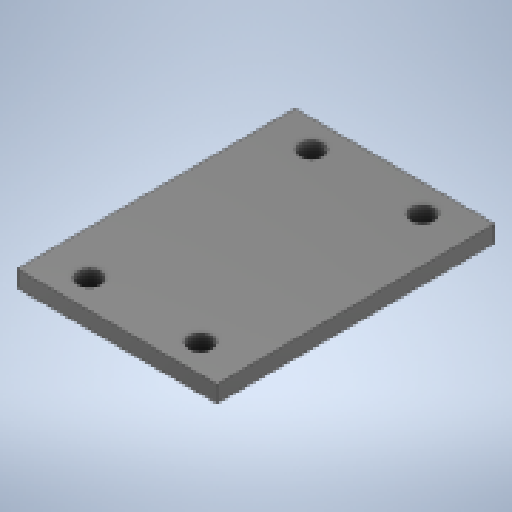
# Autodesk Inventor part: nozzle_case
Saved by Autodesk Inventor 2026.2 (Build 302298010, 298A)
## iProperties
Created: 2026-05-03
Part Number: nozzle_case
Material: ABS Plastic
Document SubType Name: Modeling
Designer: chris
Density: 1.06 g/cm^3
Appearance: Smooth - White
Author: chris
Autodesk Inventor part; units mm, degrees
ref_plane "YZ Plane" through (0, 0, 0) normal (1, 0, 0) x (0, 1, 0)
ref_plane "XZ Plane" through (0, 0, 0) normal (0, 1, 0) x (-1, 0, 0)
ref_plane "XY Plane" through (0, 0, 0) normal (0, 0, 1) x (1, 0, 0)
sketch "Sketch1" plane through (0, 0, 0) normal (0, 1, 0) x (-1, 0, 0)
  line L0 (18, 25) -> (-18, 25)
  line L1 (-18, 25) -> (-18, -25)
  line L2 (-18, -25) -> (18, -25)
  line L3 (18, -25) -> (18, 25)
  line L4 (18, 25) -> (-18, -25) construction
  line L5 (-18, 25) -> (18, -25) construction
  point P0 (0, 0)
  dimension "d0" = 36
  dimension "d1" = 50
  constraints: 12 end point, 2 midpoint, 2 parallel, 1 horizontal, 1 perpendicular
  measures "d0" distance of L2.end L1.end
  measures "d1" distance of L1.end L0.end
extrude "Extrusion1" add sketch "Sketch1" along normal blind 3
sketch "Sketch2" plane through (0, 3, 0) normal (0, 1, 0) x (1, 0, 0)
  circle A0 centre (-10, 20) radius 2.05
  circle A1 centre (10, 20) radius 2.05
  circle A2 centre (-10, -20) radius 2.05
  circle A3 centre (10, -20) radius 2.05
  point P0 (0, 0)
  dimension "d4" = 4.1
  dimension "d5" = 4.1
  dimension "d6" = 4.1
  dimension "d7" = 4.1
  dimension "d8" = 10
  dimension "d9" = 10
  dimension "d10" = 10
  dimension "d11" = 10
  dimension "d12" = 20
  dimension "d13" = 20
  dimension "d14" = 20
  dimension "d15" = 20
  constraints: 4 centre point
  measures "d4" diameter of A0
  measures "d5" diameter of A1
  measures "d6" diameter of A2
  measures "d7" diameter of A3
  measures "d8" horizontal distance of A2.centre point (0, 0)
  measures "d9" horizontal distance of A3.centre point (0, 0)
  measures "d10" horizontal distance of point (0, 0) A0.centre
  measures "d11" horizontal distance of A1.centre point (0, 0)
  measures "d12" vertical distance of A1.centre point (0, 0)
  measures "d13" vertical distance of point (0, 0) A0.centre
  measures "d14" vertical distance of point (0, 0) A2.centre
  measures "d15" vertical distance of point (0, 0) A3.centre
extrude "Extrusion2" cut sketch "Sketch2" against normal blind 3
body "Solid1"
